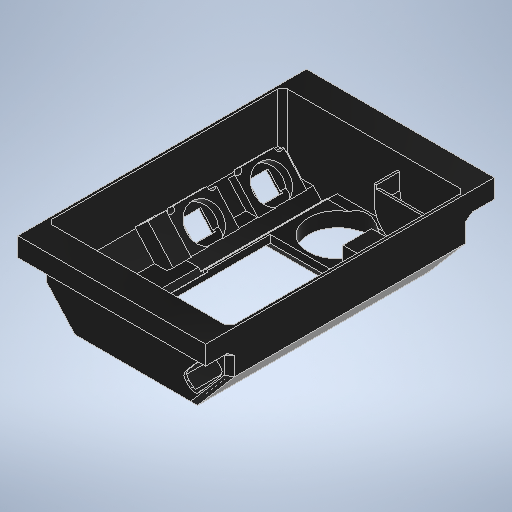
# Autodesk Inventor part: CaseTop
Saved by Autodesk Inventor 2025.2 (Build 292293000, 293)
## iProperties
Created: 2026-02-20
Part Number: CaseTop
Material: 一般
Document SubType Name: Modeling
Designer: naka6
Density: 1 g/cm^3
Appearance: ポリカーボネート - スモーク
Author: naka6
Autodesk Inventor part; units mm, degrees
ref_plane "YZ Plane" through (0, 0, 0) normal (1, 0, 0) x (0, 1, 0)
ref_plane "XZ Plane" through (0, 0, 0) normal (0, 1, 0) x (-1, 0, 0)
ref_plane "XY Plane" through (0, 0, 0) normal (0, 0, 1) x (1, 0, 0)
sketch "スケッチ1" plane through (0, 0, 0) normal (0, 0, 1) x (1, 0, 0)
  line L0 (0, 0) -> (25, 0) projected
  line L1 (25, 0) -> (25, 5) projected
  line L2 (0, 5) -> (25, 5) projected
  line L3 (0, 0) -> (0, 5) projected
  line L4 (26.3508, -9.3108) -> (30.8534, -4.0296) projected
  line L5 (-3.8505, -8.7712) -> (-2.8623, -9.8668) projected
  line L6 (-1.1891, -11.7217) -> (-2.8623, -9.8668) projected
  line L7 (-1.1891, -11.7217) -> (-0.2009, -12.8172) projected
  line L8 (5.9822, -13) -> (17.9822, -13) projected
  line L9 (32.9146, -13) -> (-6.6069, -13)
  line L10 (-6.6069, -13) -> (-6.6069, 5)
  line L11 (-6.6069, 5) -> (32.9146, 5)
  line L12 (32.9146, 5) -> (32.9146, -13)
  line L13 (31.9146, 2.3326) -> (30.7123, 3.3577) projected
  line L14 (31.9222, 2.3261) -> (31.4032, 1.7173) projected
  line L15 (-3.3792, -0.7537) -> (-5.6069, -2.7631) projected
  line L16 (-4.6007, -5.2223) -> (0.0879, -10.4201) projected
  line L17 (32.9146, -4) -> (24.3535, -14.0417)
  line L18 (-0.036, -13) -> (-6.6069, -5.7154)
  point P0 (-5.6069, -7.8692)
  point P1 (25.2416, -13)
  dimension "d0" = 0
  dimension "d1" = 0
  dimension "d2" = 0
  dimension "d26" = 1
  dimension "d27" = 1
  constraints: 12 end point, 4 parallel, 2 point on line, 1 horizontal, 1 midpoint, 1 perpendicular
  measures "d0" distance between parallel lines of L11 L2
  measures "d1" distance between parallel lines of L9 L8
  measures "d2" distance between parallel lines of L18 L6
  measures "d26" distance from line of L12 L13.start
  measures "d27" distance from line of L10 L15.end
extrude "押し出し1" add sketch "スケッチ1" along normal blind 1 contours L3 L2 L1 L0 | L0 L1 L11 L12 L17 L9 L8 L18 L7 L6 L5 L10 L3
sketch "スケッチ2" plane through (0, 0, 0) normal (0, 0, -1) x (-1, 0, 0)
  line L0 (6.6069, 5) -> (6.6069, -5.7154) projected
  line L1 (-32.9146, 5) -> (6.6069, 5) projected
  line L2 (-32.9146, -4) -> (-32.9146, 5) projected
  line L3 (0.036, -13) -> (-25.2416, -13) projected
  line L4 (-25.2416, -13) -> (-32.9146, -4) projected
  line L5 (6.6069, -5.7154) -> (0.036, -13) projected
  point P0 (0, 0)
extrude "押し出し2" add sketch "スケッチ2" along normal blind 49.75
shell "シェル1" thickness 0.6 removed faces 1 at (19.7408, 5, -15.9167)
sketch "スケッチ3" plane through (0.2308, -12.4, -49.15) normal (0, 1, 0) x (1, 0, 0)
  circle A0 centre (15.0015, -6.4) radius 0.25 projected
  circle A1 centre (8.5015, -6.4) radius 0.25 projected
  circle A2 centre (11.7515, -6.4) radius 6 projected
  line L0 (18.7692, -13.65) -> (18.7692, -44.15) construction
  line L1 (4.7692, -13.65) -> (18.7692, -13.65) construction
  line L2 (17.8672, -13.65) -> (17.8672, -44.15) construction
  line L3 (4.7692, -44.15) -> (4.7692, -13.65) construction
  line L4 (18.7692, -44.15) -> (4.7692, -44.15) construction
  circle A3 centre (11.7515, -6.4) radius 6.2
  point P0 (-0.2308, -49.15)
  dimension "d22" = 0.2
  constraints: 1 centre point
  measures "d22" radial gap between concentric circles of A2 A3
extrude "押し出し3" cut sketch "スケッチ3" against normal through all contours A0 | A1 | A2 | A3
sketch "スケッチ4" plane through (-0.036, -13, 1) normal (0, -1, 0) x (1, 0, 0)
  line L0 (19.036, -36.5) -> (19.036, -6) projected
  line L1 (5.036, -36.5) -> (19.036, -36.5) projected
  line L2 (5.036, -6) -> (5.036, -36.5) projected
  line L3 (19.036, -6) -> (5.036, -6) projected
  line L4 (19.236, -5.8) -> (19.236, -36.7)
  line L5 (19.236, -36.7) -> (4.836, -36.7)
  line L6 (4.836, -36.7) -> (4.836, -5.8)
  line L7 (4.836, -5.8) -> (19.236, -5.8)
  point P0 (0.036, -1)
  dimension "d12" = 0.2
  constraints: 8 end point, 3 other
  measures "d12" distance between parallel lines of L0 L4
extrude "押し出し4" cut sketch "スケッチ4" against normal through all contours L1 L2 L3 L0 | L4 L5 L6 L7
sketch "スケッチ5" plane through (0.2308, -12.4, -49.15) normal (0, 1, 0) x (1, 0, 0)
  line L0 (24.7339, 0) -> (24.7339, -49.55) projected
  line L1 (24.7339, 0) -> (0, 0) projected
  line L2 (0, 0) -> (0, -49.55) projected
  line L3 (0, -49.55) -> (24.7339, -49.55) projected
  line L4 (18.9692, -13.45) -> (4.5692, -13.45) projected
  line L5 (4.5692, -13.45) -> (4.5692, -44.35) projected
  line L6 (4.5692, -44.35) -> (18.9692, -44.35) projected
  line L7 (18.9692, -44.35) -> (18.9692, -13.45) projected
  circle A0 centre (11.7515, -6.4) radius 6.2 projected
  line L8 (25.0108, 0.6) -> (25.0108, -50.15) projected
  line L9 (-0.2668, -50.15) -> (25.0108, -50.15) projected
  line L10 (-0.2668, 0.6) -> (-0.2668, -50.15) projected
  line L11 (25.0108, 0.6) -> (-0.2668, 0.6) projected
  point P0 (-0.2308, -49.15)
extrude "押し出し5" add sketch "スケッチ5" along normal blind 2.5 contours L0 L3 L2 L1
chamfer "面取り1" distance 2.5 distance2 1.5 3 edges at (4.8, -13, -20.25) (12, -13, -4.8) (19.2, -13, -20.25) measured on face at (4.3, -13, -20.25) measured on face at (12, -13, -4.3) measured on face at (19.7, -13, -20.25)
chamfer "面取り3" distance 0.6 distance2 1.5 3 edges at (3.55, -13, -35.7) (12, -13, -35.7) (20.45, -13, -35.7) measured on face at (3.55, -13, -36.2) measured on face at (20.45, -13, -36.2) measured on face at (12, -13, -36.2)
sketch "スケッチ7" plane through (-0.036, -13, -49.75) normal (-0.7425471, -0.6697938, 0) x (0, 0, 1)
  line L0 (23.2879, 7.2327) -> (19.4879, 7.2327) projected
  line L1 (19.4879, 7.2327) -> (19.4879, 3.4327) projected
  line L2 (19.4879, 3.4327) -> (23.2879, 3.4327) projected
  line L3 (23.2879, 3.4327) -> (23.2879, 7.2327) projected
  circle A0 centre (21.3879, 5.3327) radius 0.9 projected
  line L4 (9.1216, 7.2327) -> (5.3216, 7.2327) projected
  line L5 (5.3216, 7.2327) -> (5.3216, 3.4327) projected
  line L6 (5.3216, 3.4327) -> (9.1216, 3.4327) projected
  line L7 (9.1216, 3.4327) -> (9.1216, 7.2327) projected
  circle A1 centre (7.2216, 5.3327) radius 0.9 projected
  line L8 (23.4879, 7.4327) -> (19.2879, 7.4327)
  line L9 (19.2879, 7.4327) -> (19.2879, 3.2327)
  line L10 (19.2879, 3.2327) -> (23.4879, 3.2327)
  line L11 (23.4879, 3.2327) -> (23.4879, 7.4327)
  line L12 (9.3216, 7.4327) -> (5.1216, 7.4327)
  line L13 (5.1216, 7.4327) -> (5.1216, 3.2327)
  line L14 (5.1216, 3.2327) -> (9.3216, 3.2327)
  line L15 (9.3216, 3.2327) -> (9.3216, 7.4327)
  point P0 (49.75, 9.629)
  dimension "d30" = 0.2
  dimension "d31" = 0.2
  constraints: 16 end point, 6 other
  measures "d30" distance between parallel lines of L3 L11
  measures "d31" distance between parallel lines of L7 L15
sketch "スケッチ8" plane through (24.9647, -12.4, -49.15) normal (1, 0, 0) x (0, 0, -1)
  line L0 (0, 0) -> (-49.55, 0) projected
  line L1 (0, 2.5) -> (0, 0) projected
  line L2 (-49.55, 2.5) -> (0, 2.5) projected
  line L3 (-49.55, 0) -> (-49.55, 2.5) projected
  point P0 (-49.15, 12.4)
extrude "押し出し8" add sketch "スケッチ8" along normal up to surface surface through (24.785, -12.6107, 0) normal (0.7609777, -0.6487781, 0)
sketch "スケッチ9" plane through (0.2308, -12.4, 0.4) normal (-1, 0, 0) x (0, 0, 1)
  line L0 (-49.55, 0) -> (0, 0) projected
  line L1 (0, 2.5) -> (0, 0) projected
  line L2 (-49.55, 2.5) -> (0, 2.5) projected
  line L3 (-49.55, 0) -> (-49.55, 2.5) projected
  point P0 (-0.4, 12.4)
extrude "押し出し9" add sketch "スケッチ9" along normal up to surface surface through (-6.1613, -5.3136, 0) normal (-0.7425471, -0.6697938, 0)
extrude "押し出し10" cut sketch "スケッチ7" against normal through all contours L3 L2 L1 L0 | A0 | L7 L6 L5 L4 | A1 | L11 L10 L9 L8 | L15 L14 L13 L12
sketch "スケッチ10" plane through (-0.036, -13, -49.75) normal (-0.7425471, -0.6697938, 0) x (0, 0, 1)
  arc A0 (41.0449, 0.0976) -> (43.25, 1.686) centre (40.65, 2.9706) ccw projected
  arc A1 (40.8745, 0.2462) -> (41.0449, 0.0976) centre (41.0245, 0.2462) ccw projected
  arc A2 (40.8745, 0.2462) -> (40.4255, 0.2462) centre (40.65, 0.2463) ccw projected
  line L0 (9.3216, 3.2327) -> (5.1216, 3.2327) projected
  line L1 (5.1216, 3.2327) -> (5.1216, 7.4327) projected
  line L2 (5.1216, 7.4327) -> (9.3216, 7.4327) projected
  line L3 (9.3216, 7.4327) -> (9.3216, 3.2327) projected
  line L4 (23.4879, 3.2327) -> (19.2879, 3.2327) projected
  line L5 (19.2879, 3.2327) -> (19.2879, 7.4327) projected
  line L6 (19.2879, 7.4327) -> (23.4879, 7.4327) projected
  line L7 (23.4879, 7.4327) -> (23.4879, 3.2327) projected
  line L8 (0, 0) -> (50.75, 0) projected
  line L9 (50.75, 9.8102) -> (50.75, 0) projected
  line L10 (0, 9.8102) -> (50.75, 9.8102) projected
  line L11 (0, 0) -> (0, 9.8102) projected
  arc A3 (40.2551, 0.0976) -> (40.4255, 0.2462) centre (40.2755, 0.2462) ccw projected
  arc A4 (38.05, 1.686) -> (40.2551, 0.0976) centre (40.65, 2.9706) ccw projected
  line L12 (43.25, 1.686) -> (43.25, 4.2551) projected
  arc A5 (43.25, 4.2551) -> (41.0449, 5.8435) centre (40.65, 2.9706) ccw projected
  line L13 (38.05, 4.2551) -> (38.05, 1.686) projected
  arc A6 (40.2551, 5.8435) -> (38.05, 4.2551) centre (40.65, 2.9706) ccw projected
  arc A7 (40.4255, 5.6949) -> (40.2551, 5.8435) centre (40.2755, 5.6949) ccw projected
  arc A8 (40.4255, 5.6949) -> (40.8745, 5.6949) centre (40.65, 5.6949) ccw projected
  arc A9 (41.0449, 5.8435) -> (40.8745, 5.6949) centre (41.0245, 5.6949) ccw projected
  point P0 (49.75, 9.629)
  point P1 (40.4255, 0.2462)
extrude "押し出し11" cut sketch "スケッチ10" against normal through all contours A1 A2 A3 A4 L13 A6 A7 A8 A9 A5 L12 A0
sketch "スケッチ11" plane through (-6.0069, -5.4848, 0.4) normal (0.7425471, 0.6697938, 0) x (0, 0, -1)
  line L0 (6.9, -5.3245) -> (6.9, -7.8936) projected
  arc A0 (6.9, -7.8936) -> (9.1051, -9.482) centre (9.5, -6.609) ccw projected
  arc A1 (9.1051, -9.482) -> (9.2755, -9.3334) centre (9.1255, -9.3334) ccw projected
  arc A2 (9.7245, -9.3334) -> (9.2755, -9.3334) centre (9.5, -9.3333) ccw projected
  arc A3 (9.7245, -9.3334) -> (9.8949, -9.482) centre (9.8745, -9.3334) ccw projected
  arc A4 (9.8949, -9.482) -> (12.1, -7.8936) centre (9.5, -6.609) ccw projected
  line L1 (12.1, -7.8936) -> (12.1, -5.3245) projected
  arc A5 (12.1, -5.3245) -> (9.8949, -3.736) centre (9.5, -6.609) ccw projected
  arc A6 (9.8949, -3.736) -> (9.7245, -3.8846) centre (9.8745, -3.8846) ccw projected
  arc A7 (9.2755, -3.8847) -> (9.7245, -3.8846) centre (9.5, -3.8847) ccw projected
  arc A8 (9.2755, -3.8847) -> (9.1051, -3.736) centre (9.1255, -3.8846) ccw projected
  arc A9 (9.1051, -3.736) -> (6.9, -5.3245) centre (9.5, -6.609) ccw projected
  line L2 (40.8284, -6.3469) -> (45.0284, -6.3469) projected
  line L3 (45.0284, -6.3469) -> (45.0284, -2.1469) projected
  line L4 (45.0284, -2.1469) -> (40.8284, -2.1469) projected
  line L5 (40.8284, -2.1469) -> (40.8284, -6.3469) projected
  line L6 (26.6621, -6.3469) -> (30.8621, -6.3469) projected
  line L7 (30.8621, -6.3469) -> (30.8621, -2.1469) projected
  line L8 (30.8621, -2.1469) -> (26.6621, -2.1469) projected
  line L9 (26.6621, -2.1469) -> (26.6621, -6.3469) projected
  line L10 (50.15, -9.5796) -> (-0.6, -9.5796) projected
  line L11 (-0.6, 0.2306) -> (-0.6, -9.5796) projected
  line L12 (50.15, 0.2306) -> (-0.6, 0.2306) projected
  line L13 (50.15, -9.5796) -> (50.15, 0.2306) projected
  circle A10 centre (42.9284, -4.2469) radius 3.5 projected
  line L14 (23.2621, -9.0398) -> (23.2621, 0.546) projected
  line L15 (23.2621, 0.546) -> (23.9692, 1.2531) projected
  line L16 (23.9692, 1.2531) -> (33.555, 1.2531) projected
  line L17 (33.555, 1.2531) -> (34.2621, 0.546) projected
  line L18 (34.2621, 0.546) -> (34.2621, -9.0398) projected
  line L19 (34.2621, -9.0398) -> (33.555, -9.7469) projected
  line L20 (33.555, -9.7469) -> (23.9692, -9.7469) projected
  line L21 (23.9692, -9.7469) -> (23.2621, -9.0398) projected
  circle A11 centre (28.7621, -4.2469) radius 3.5 projected
  circle A12 centre (33.1621, -8.6469) radius 0.7 projected
  circle A13 centre (24.3621, -8.6469) radius 0.7 projected
  circle A14 centre (24.3621, 0.1531) radius 0.7 projected
  circle A15 centre (33.1621, 0.1531) radius 0.7 projected
  line L22 (37.4284, -9.0398) -> (37.4284, 0.546) projected
  line L23 (37.4284, 0.546) -> (38.1355, 1.2531) projected
  line L24 (38.1355, 1.2531) -> (47.7213, 1.2531) projected
  line L25 (47.7213, 1.2531) -> (48.4284, 0.546) projected
  line L26 (48.4284, 0.546) -> (48.4284, -9.0398) projected
  line L27 (48.4284, -9.0398) -> (47.7213, -9.7469) projected
  line L28 (47.7213, -9.7469) -> (38.1355, -9.7469) projected
  line L29 (38.1355, -9.7469) -> (37.4284, -9.0398) projected
  circle A16 centre (42.9284, -4.2469) radius 3.5 projected
  circle A17 centre (47.3284, -8.6469) radius 0.7 projected
  circle A18 centre (38.5284, -8.6469) radius 0.7 projected
  circle A19 centre (38.5284, 0.1531) radius 0.7 projected
  circle A20 centre (47.3284, 0.1531) radius 0.7 projected
  line L30 (22.4, 0.2429) -> (22.4, -10.7571) projected
  line L31 (22.4, -10.7571) -> (0.4, -10.7571) projected
  line L32 (0.4, -10.7571) -> (0.4, 0.2429) projected
  line L33 (0.4, 0.2429) -> (22.4, 0.2429) projected
  line L34 (19.8649, -8.2571) -> (20.8649, -8.2571) projected
  arc A21 (19.8649, -8.2571) -> (19.8649, -10.2571) centre (19.8649, -9.2571) ccw projected
  line L35 (20.8649, -10.2571) -> (19.8649, -10.2571) projected
  arc A22 (20.8649, -10.2571) -> (20.8649, -8.2571) centre (20.8649, -9.2571) ccw projected
  line L36 (19.8649, -4.2571) -> (20.8649, -4.2571) projected
  arc A23 (19.8649, -4.2571) -> (19.8649, -6.2571) centre (19.8649, -5.2571) ccw projected
  line L37 (20.8649, -6.2571) -> (19.8649, -6.2571) projected
  arc A24 (20.8649, -6.2571) -> (20.8649, -4.2571) centre (20.8649, -5.2571) ccw projected
  line L38 (1.6, -0.2571) -> (2.6, -0.2571) projected
  arc A25 (1.6, -0.2571) -> (1.6, -2.2571) centre (1.6, -1.2571) ccw projected
  line L39 (2.6, -2.2571) -> (1.6, -2.2571) projected
  arc A26 (2.6, -2.2571) -> (2.6, -0.2571) centre (2.6, -1.2571) ccw projected
  line L40 (1.6, -8.2571) -> (2.6, -8.2571) projected
  arc A27 (1.6, -8.2571) -> (1.6, -10.2571) centre (1.6, -9.2571) ccw projected
  line L41 (2.6, -10.2571) -> (1.6, -10.2571) projected
  arc A28 (2.6, -10.2571) -> (2.6, -8.2571) centre (2.6, -9.2571) ccw projected
  line L42 (24.1349, -9.3469) -> (33.3893, -9.3469)
  line L43 (33.3893, -9.3469) -> (33.8621, -8.8741)
  line L44 (33.8621, -8.8741) -> (33.8621, 0.3803)
  line L45 (33.8621, 0.3803) -> (33.3893, 0.8531)
  line L46 (33.3893, 0.8531) -> (24.1349, 0.8531)
  line L47 (24.1349, 0.8531) -> (23.6621, 0.3803)
  line L48 (23.6621, 0.3803) -> (23.6621, -8.8741)
  line L49 (23.6621, -8.8741) -> (24.1349, -9.3469)
  circle A29 centre (24.3621, -8.6469) radius 0.9
  circle A30 centre (33.1621, -8.6469) radius 0.9
  circle A31 centre (33.1621, 0.1531) radius 0.9
  circle A32 centre (24.3621, 0.1531) radius 0.9
  circle A33 centre (28.7621, -4.2469) radius 3.7
  line L50 (38.3012, -9.3469) -> (47.5556, -9.3469)
  line L51 (47.5556, -9.3469) -> (48.0284, -8.8741)
  line L52 (48.0284, -8.8741) -> (48.0284, 0.3803)
  line L53 (48.0284, 0.3803) -> (47.5556, 0.8531)
  line L54 (47.5556, 0.8531) -> (38.3012, 0.8531)
  line L55 (38.3012, 0.8531) -> (37.8284, 0.3803)
  line L56 (37.8284, 0.3803) -> (37.8284, -8.8741)
  line L57 (37.8284, -8.8741) -> (38.3012, -9.3469)
  circle A34 centre (38.5284, -8.6469) radius 0.9
  circle A35 centre (38.5284, 0.1531) radius 0.9
  circle A36 centre (47.3284, 0.1531) radius 0.9
  circle A37 centre (47.3284, -8.6469) radius 0.9
  circle A38 centre (42.9284, -4.2469) radius 3.7
  line L58 (22.4, -10.7571) -> (18.6046, -10.7571)
  line L59 (18.6046, -10.7571) -> (18.6046, 0.2429)
  line L60 (18.6046, 0.2429) -> (22.4, 0.2429)
  line L61 (22.4, 0.2429) -> (22.4, -10.7571)
  line L62 (0.4, -10.7571) -> (3.8976, -10.7571)
  line L63 (3.8976, -10.7571) -> (3.8976, -7.8936)
  line L64 (3.8976, -7.8936) -> (0.4, -7.8936)
  line L65 (0.4, -7.8936) -> (0.4, -10.7571)
  line L66 (0.4, 0.0494) -> (3.8976, 0.0494)
  line L67 (3.8976, 0.0494) -> (3.8976, -2.666)
  line L68 (3.8976, -2.666) -> (0.4, -2.666)
  line L69 (0.4, -2.666) -> (0.4, 0.0494)
  point P0 (46.7627, -9.3469)
  point P1 (48.0284, -8.0812)
  point P2 (48.0284, -0.4126)
  point P3 (46.4318, 0.2306)
  point P4 (39.4251, 0.2306)
  point P5 (37.8284, -0.4126)
  point P6 (37.8284, -8.0812)
  point P7 (39.0941, -9.3469)
  point P8 (25.2587, 0.2306)
  point P9 (23.6621, -0.4126)
  point P10 (23.6621, -8.0812)
  point P11 (24.9278, -9.3469)
  point P12 (32.5964, -9.3469)
  point P13 (33.8621, -8.0812)
  point P14 (33.8621, -0.4126)
  point P15 (32.2654, 0.2306)
  point P16 (22.4, -9.5796)
  point P17 (22.4, 0.2306)
  point P18 (18.6046, 0.2306)
  point P19 (18.6046, -9.5796)
  point P20 (3.8976, -9.5796)
  point P21 (0.4, -7.8936)
  point P22 (0.4, -9.5796)
  point P23 (0.4, -2.666)
  dimension "d42" = 0.4
  dimension "d43" = 0.2
  dimension "d44" = 0.2
  dimension "d45" = 0.2
  dimension "d46" = 0.2
  dimension "d47" = 0.2
  dimension "d48" = 0.4
  dimension "d49" = 0.2
  dimension "d50" = 0.2
  dimension "d51" = 0.2
  dimension "d52" = 0.2
  dimension "d53" = 0.2
  constraints: 56 end point, 10 centre point, 6 parallel, 3 horizontal, 3 perpendicular, 2 point on line, 14 other
  measures "d42" distance between parallel lines of L20 L42
  measures "d43" radial gap between concentric circles of A13 A29
  measures "d44" radial gap between concentric circles of A12 A30
  measures "d45" radial gap between concentric circles of A15 A31
  measures "d46" radial gap between concentric circles of A14 A32
  measures "d47" radial gap between concentric circles of A11 A33
  measures "d48" distance between parallel lines of L28 L50
  measures "d49" radial gap between concentric circles of A18 A34
  measures "d50" radial gap between concentric circles of A19 A35
  measures "d51" radial gap between concentric circles of A20 A36
  measures "d52" radial gap between concentric circles of A17 A37
  measures "d53" radial gap between concentric circles of A16 A38
extrude "押し出し12" add sketch "スケッチ11" along normal blind 1.92 contours L10 A22 L34 A21 L59 L12 L30 | L52 A37 L50 A34 L56 A35 L12 A36 | L10 A21 L34 A22 | A32 L12 A31 L44 A30 L42 A29 L48 | L10 A28 L40 A27 L32 L64 L63 | L66 L67 L68 L32 | L10 A27 L40 A28 | L36 A24 L37 A23 | L38 A26 L39 A25
sketch "スケッチ12" plane through (-4.5812, -4.1988, 0.4) normal (0.7425471, 0.6697938, 0) x (0, 0, -1)
  line L0 (22.4, -7.6779) -> (18.6046, -7.6779) projected
  line L1 (22.4, -7.6779) -> (22.4, 0.2306) projected
  line L2 (22.4, 0.2306) -> (18.6046, 0.2306) projected
  line L3 (18.6046, 0.2306) -> (18.6046, -7.6779) projected
  line L4 (3.8976, 0.0494) -> (0.4, 0.0494) projected
  line L5 (0.4, 0.0494) -> (0.4, -2.666) projected
  line L6 (0.4, -2.666) -> (3.8976, -2.666) projected
  line L7 (3.8976, -2.666) -> (3.8976, 0.0494) projected
  point P0 (0.4, 0.0494)
extrude "押し出し13" add sketch "スケッチ12" along normal blind 1.8
sketch "スケッチ13" plane through (32.3146, 5, 0.4) normal (0, 0, -1) x (-1, 0, 0)
  line L0 (28.2057, -15.8469) -> (27.3146, -15.0431) projected
  line L1 (35.5734, -7.6788) -> (28.2057, -15.8469) projected
  line L2 (27.3146, -15.0431) -> (27.156, -14.9)
  line L3 (5.2186, -14.9) -> (34.3389, -14.9) projected
  point P0 (32.3146, -5)
  point P1 (29.0597, -14.9)
  constraints: 2 end point, 1 collinear, 1 point on line
extrude "押し出し14" cut sketch "スケッチ13" along normal blind 23
sketch "スケッチ14" plane through (-6.0069, 5, -49.15) normal (0, 0, 1) x (1, 0, 0)
  line L0 (0.4, -7.7631) -> (1.0698, -8.5057)
  line L1 (2.6276, -5.7537) -> (0.4, -7.7631)
  line L2 (7.7677, -15.9311) -> (1.0698, -8.5057)
  line L3 (7.7677, -15.9311) -> (9.9954, -13.9218)
  line L4 (3.9826, -14.9) -> (33.1029, -14.9)
  line L5 (6.6742, -15.1668) -> (7.6119, -16.2063)
  line L6 (5.8059, -17.8172) -> (9.04, -14.9)
  line L7 (6.6742, -15.1668) -> (6.4336, -14.9)
  line L8 (8.4375, -16.6737) -> (7.7677, -15.9311)
  line L9 (10.6652, -14.6643) -> (8.4375, -16.6737)
  line L10 (8.4375, -16.6737) -> (6.9671, -18)
  line L11 (5.9708, -18) -> (31.2484, -18)
  line L12 (7.6029, -16.1963) -> (8.2148, -16.8746)
  point P0 (6.0069, -5)
  point P1 (7.6029, -16.1963)
  point P2 (10.4039, -14.9)
extrude "押し出し15" cut sketch "スケッチ14" along normal blind 27
sketch "スケッチ15" plane through (32.3146, 5, 0.4) normal (0, 0, -1) x (-1, 0, 0)
  line L0 (12.0704, -16.3714) -> (11.5514, -15.7627) projected
  line L1 (0.9114, -3.2827) -> (11.5514, -15.7627) projected
  line L2 (13.2804, -15.3399) -> (12.078, -16.365) projected
  line L3 (13.2804, -15.3399) -> (13.7964, -14.9)
  line L4 (27.9176, -14.9) -> (5.2186, -14.9) projected
  line L5 (12.078, -16.365) -> (12.0704, -16.3714)
  point P0 (32.3146, -5)
  point P1 (10.8159, -14.9)
  constraints: 4 end point, 1 collinear, 1 point on line
extrude "押し出し16" cut sketch "スケッチ15" along normal blind 25.25
sketch "スケッチ16" plane through (0, 0, 1) normal (0, 0, 1) x (1, 0, 0)
  line L0 (26.3508, -9.3108) -> (30.8534, -4.0296) projected
  arc A0 (24.9411, -9.423) -> (26.3508, -9.3108) centre (25.5899, -8.662) ccw projected
  line L1 (24.0203, -8.638) -> (24.9411, -9.423) projected
  arc A1 (30.8534, -4.0296) -> (30.7412, -2.6198) centre (30.0924, -3.3808) ccw projected
  line L2 (30.7412, -2.6198) -> (29.8204, -1.8348) projected
  arc A2 (29.8204, -1.8348) -> (28.4106, -1.947) centre (29.1716, -2.5958) ccw projected
  line L3 (28.4106, -1.947) -> (25.9323, -4.854) projected
  line L4 (25.8998, -4.892) -> (23.9081, -7.2282) projected
  arc A3 (23.9081, -7.2282) -> (24.0203, -8.638) centre (24.6691, -7.877) ccw projected
  line L5 (25.6716, -4.6974) -> (23.6798, -7.0336)
  arc A4 (23.6798, -7.0336) -> (23.8257, -8.8663) centre (24.6691, -7.877) ccw
  line L6 (23.8257, -8.8663) -> (24.7464, -9.6513)
  arc A5 (24.7464, -9.6513) -> (26.5791, -9.5054) centre (25.5899, -8.662) ccw
  line L7 (26.5791, -9.5054) -> (31.0817, -4.2242)
  arc A6 (31.0817, -4.2242) -> (30.9358, -2.3916) centre (30.0924, -3.3808) ccw
  line L8 (30.9358, -2.3916) -> (30.015, -1.6065)
  arc A7 (30.015, -1.6065) -> (28.1823, -1.7524) centre (29.1716, -2.5958) ccw
  line L9 (28.1823, -1.7524) -> (25.704, -4.6593)
  line L10 (25.6716, -4.6974) -> (25.704, -4.6593)
  point P0 (0, 0)
  dimension "d64" = 0.3
  constraints: 12 end point, 8 point on circle, 4 centre point, 1 collinear, 8 other
  measures "d64" distance between parallel lines of L4 L5
extrude "押し出し17" cut sketch "スケッチ16" against normal blind 8
sketch "スケッチ17" plane through (32.3146, -3.7789, -49.15) normal (-0.7609777, 0.6487781, 0) x (0, 0, 1)
  line L0 (0, 0) -> (49.55, 0) projected
  line L1 (0, -8.0437) -> (49.55, -8.0437) projected
  arc A0 (48.1, 3.5912) -> (47.31, 4.3912) centre (47.3, 3.5912) ccw projected
  line L2 (47.31, 4.3912) -> (47.31, 3.0112) projected
  arc A1 (45.71, 3.0112) -> (47.31, 3.0112) centre (46.51, 3.0112) ccw projected
  line L3 (45.71, 3.0112) -> (45.71, 4.3912) projected
  line L4 (45.71, 4.3912) -> (44.77, 4.3912) projected
  line L5 (44.77, 4.3912) -> (44.77, 3.0112) projected
  arc A2 (43.17, 3.0112) -> (44.77, 3.0112) centre (43.97, 3.0112) ccw projected
  line L6 (43.17, 3.0112) -> (43.17, 4.3912) projected
  line L7 (43.17, 4.3912) -> (42.23, 4.3912) projected
  line L8 (42.23, 4.3912) -> (42.23, 3.0112) projected
  arc A3 (40.63, 3.0112) -> (42.23, 3.0112) centre (41.43, 3.0112) ccw projected
  line L9 (40.63, 3.0112) -> (40.63, 4.3912) projected
  line L10 (40.63, 4.3912) -> (39.69, 4.3912) projected
  line L11 (39.69, 4.3912) -> (39.69, 3.0112) projected
  arc A4 (38.09, 3.0112) -> (39.69, 3.0112) centre (38.89, 3.0112) ccw projected
  line L12 (38.09, 3.0112) -> (38.09, 4.3912) projected
  line L13 (38.09, 4.3912) -> (37.15, 4.3912) projected
  line L14 (37.15, 4.3912) -> (37.15, 3.0112) projected
  arc A5 (35.55, 3.0112) -> (37.15, 3.0112) centre (36.35, 3.0112) ccw projected
  line L15 (35.55, 3.0112) -> (35.55, 4.3912) projected
  line L16 (35.55, 4.3912) -> (34.61, 4.3912) projected
  line L17 (34.61, 4.3912) -> (34.61, 3.0112) projected
  arc A6 (33.01, 3.0112) -> (34.61, 3.0112) centre (33.81, 3.0112) ccw projected
  line L18 (33.01, 3.0112) -> (33.01, 4.3912) projected
  line L19 (33.01, 4.3912) -> (32.07, 4.3912) projected
  line L20 (32.07, 4.3912) -> (32.07, 3.0112) projected
  arc A7 (30.47, 3.0112) -> (32.07, 3.0112) centre (31.27, 3.0112) ccw projected
  line L21 (30.47, 3.0112) -> (30.47, 4.3912) projected
  line L22 (30.47, 4.3912) -> (29.53, 4.3912) projected
  line L23 (29.53, 4.3912) -> (29.53, 3.0112) projected
  arc A8 (27.93, 3.0112) -> (29.53, 3.0112) centre (28.73, 3.0112) ccw projected
  line L24 (27.93, 3.0112) -> (27.93, 4.3912) projected
  line L25 (27.93, 4.3912) -> (26.99, 4.3912) projected
  line L26 (26.99, 4.3912) -> (26.99, 3.0112) projected
  arc A9 (25.39, 3.0112) -> (26.99, 3.0112) centre (26.19, 3.0112) ccw projected
  line L27 (25.39, 3.0112) -> (25.39, 4.3912) projected
  arc A10 (25.39, 4.3912) -> (24.6, 3.5912) centre (25.4, 3.5912) ccw projected
  line L28 (24.6, 3.5912) -> (24.6, -12.8088) projected
  arc A11 (24.6, -12.8088) -> (25.39, -13.6087) centre (25.4, -12.8088) ccw projected
  line L29 (25.39, -13.6087) -> (25.39, -12.2288) projected
  arc A12 (26.99, -12.2288) -> (25.39, -12.2288) centre (26.19, -12.2288) ccw projected
  line L30 (26.99, -12.2288) -> (26.99, -13.6088) projected
  line L31 (26.99, -13.6088) -> (27.93, -13.6088) projected
  line L32 (27.93, -13.6088) -> (27.93, -12.2288) projected
  arc A13 (29.53, -12.2288) -> (27.93, -12.2288) centre (28.73, -12.2288) ccw projected
  line L33 (29.53, -12.2288) -> (29.53, -13.6088) projected
  line L34 (29.53, -13.6088) -> (30.47, -13.6088) projected
  line L35 (30.47, -13.6088) -> (30.47, -12.2288) projected
  arc A14 (32.07, -12.2288) -> (30.47, -12.2288) centre (31.27, -12.2288) ccw projected
  line L36 (32.07, -12.2288) -> (32.07, -13.6088) projected
  line L37 (32.07, -13.6088) -> (33.01, -13.6088) projected
  line L38 (33.01, -13.6088) -> (33.01, -12.2288) projected
  arc A15 (34.61, -12.2288) -> (33.01, -12.2288) centre (33.81, -12.2288) ccw projected
  line L39 (34.61, -12.2288) -> (34.61, -13.6088) projected
  line L40 (34.61, -13.6088) -> (35.55, -13.6088) projected
  line L41 (35.55, -13.6088) -> (35.55, -12.2288) projected
  arc A16 (37.15, -12.2288) -> (35.55, -12.2288) centre (36.35, -12.2288) ccw projected
  line L42 (37.15, -12.2288) -> (37.15, -13.6088) projected
  line L43 (37.15, -13.6088) -> (38.09, -13.6088) projected
  line L44 (38.09, -13.6088) -> (38.09, -12.2288) projected
  arc A17 (39.69, -12.2288) -> (38.09, -12.2288) centre (38.89, -12.2288) ccw projected
  line L45 (39.69, -12.2288) -> (39.69, -13.6088) projected
  line L46 (39.69, -13.6088) -> (40.63, -13.6088) projected
  line L47 (40.63, -13.6088) -> (40.63, -12.2288) projected
  arc A18 (42.23, -12.2288) -> (40.63, -12.2288) centre (41.43, -12.2288) ccw projected
  line L48 (42.23, -12.2288) -> (42.23, -13.6088) projected
  line L49 (42.23, -13.6088) -> (43.17, -13.6088) projected
  line L50 (43.17, -13.6088) -> (43.17, -12.2288) projected
  arc A19 (44.77, -12.2288) -> (43.17, -12.2288) centre (43.97, -12.2288) ccw projected
  line L51 (44.77, -12.2288) -> (44.77, -13.6088) projected
  line L52 (44.77, -13.6088) -> (45.71, -13.6088) projected
  line L53 (45.71, -13.6088) -> (45.71, -12.2288) projected
  arc A20 (47.31, -12.2288) -> (45.71, -12.2288) centre (46.51, -12.2288) ccw projected
  line L54 (47.31, -12.2288) -> (47.31, -13.6087) projected
  arc A21 (47.31, -13.6087) -> (48.1, -12.8088) centre (47.3, -12.8088) ccw projected
  line L55 (48.1, -12.8088) -> (48.1, 3.5912) projected
  arc A22 (46.8, -9.4288) -> (46.8, -8.4288) centre (46.8, -8.9288) ccw projected
  line L56 (46.8, -9.4288) -> (46.1, -9.4288) projected
  arc A23 (46.1, -8.4288) -> (46.1, -9.4288) centre (46.1, -8.9288) ccw projected
  line L57 (46.1, -8.4288) -> (46.8, -8.4288) projected
  line L58 (43.2, -9.4288) -> (42.5, -9.4288) projected
  arc A24 (42.5, -8.4288) -> (42.5, -9.4288) centre (42.5, -8.9288) ccw projected
  line L59 (42.5, -8.4288) -> (43.2, -8.4288) projected
  arc A25 (43.2, -9.4288) -> (43.2, -8.4288) centre (43.2, -8.9288) ccw projected
  line L60 (43.2, -0.7888) -> (42.5, -0.7888) projected
  arc A26 (42.5, 0.2112) -> (42.5, -0.7888) centre (42.5, -0.2888) ccw projected
  line L61 (42.5, 0.2112) -> (43.2, 0.2112) projected
  arc A27 (43.2, -0.7888) -> (43.2, 0.2112) centre (43.2, -0.2888) ccw projected
  circle A28 centre (39.31, 0.7612) radius 0.6 projected
  circle A29 centre (37.7171, 0.7612) radius 0.6 projected
  circle A30 centre (36.1243, 0.7612) radius 0.6 projected
  circle A31 centre (34.5314, 0.7612) radius 0.6 projected
  circle A32 centre (32.9386, 0.7612) radius 0.6 projected
  circle A33 centre (31.3457, 0.7612) radius 0.6 projected
  circle A34 centre (29.7529, 0.7612) radius 0.6 projected
  circle A35 centre (28.16, 0.7612) radius 0.6 projected
  arc A36 (46.8, -0.7888) -> (46.8, 0.2112) centre (46.8, -0.2888) ccw projected
  line L62 (46.8, -0.7888) -> (46.1, -0.7888) projected
  arc A37 (46.1, 0.2112) -> (46.1, -0.7888) centre (46.1, -0.2888) ccw projected
  line L63 (46.1, 0.2112) -> (46.8, 0.2112) projected
  line L64 (24.6, 0) -> (26.99, 0)
  line L65 (26.99, 0) -> (26.99, -3.7543)
  line L66 (26.99, -3.7543) -> (24.6, -3.7543)
  line L67 (24.6, -3.7543) -> (24.6, 0)
  point P0 (49.15, -18.0893)
  point P1 (24.6, -3.7543)
  constraints: 8 end point, 2 parallel, 2 point on line, 1 horizontal, 1 perpendicular
extrude "押し出し18" add sketch "スケッチ17" along normal blind 4 contours L0 L65 L66 L28
sketch "スケッチ18" plane through (0.2308, -9.9, -49.15) normal (0, 1, 0) x (1, 0, 0)
  line L0 (18.2874, -49.55) -> (18.2874, -44.35) projected
  line L1 (18.2874, -44.35) -> (4.9279, -44.35) projected
  line L2 (4.9279, -44.35) -> (4.9279, -49.55) projected
  line L3 (18.2874, -49.55) -> (4.9279, -49.55) projected
  circle A0 centre (11.7515, -6.4) radius 6.2 projected
  line L4 (24.9624, -49.55) -> (24.9624, -42.15) projected
  line L5 (24.9624, -42.15) -> (25.7558, -42.15) projected
  line L6 (25.7558, -42.15) -> (25.7558, -49.55) projected
  line L7 (26.8653, -49.55) -> (25.7558, -49.55) projected
  line L8 (26.8653, 0) -> (26.8653, -49.55) projected
  line L9 (4.1662, 0) -> (26.8653, 0) projected
  line L10 (4.1662, 0) -> (4.1662, -26.55) projected
  line L11 (4.1662, -26.55) -> (4.5692, -26.55) projected
  line L12 (4.5692, -26.55) -> (4.5692, -13.45) projected
  line L13 (4.5692, -13.45) -> (18.9692, -13.45) projected
  line L14 (18.9692, -13.45) -> (18.9692, -24.3) projected
  line L15 (18.9692, -24.3) -> (21.268, -24.3) projected
  line L16 (21.268, -24.3) -> (21.268, -49.55) projected
  line L17 (24.9624, -49.55) -> (21.268, -49.55) projected
  line L18 (26.8653, -12.7392) -> (19.1904, -12.7392)
  line L19 (19.1904, -12.7392) -> (19.1904, -6.7025)
  line L20 (19.1904, -6.7025) -> (26.8653, -6.7025)
  line L21 (26.8653, -6.7025) -> (26.8653, -12.7392)
  point P0 (-0.2308, -49.15)
  point P1 (26.8653, -6.7025)
  constraints: 8 end point, 2 parallel, 1 horizontal, 1 perpendicular, 1 point on line
extrude "押し出し19" add sketch "スケッチ18" along normal blind 5 contours L3 L2 L1 L0 | L18 L19 L20 L8
sketch "スケッチ19" plane through (-6.0069, 5, -49.15) normal (0, 0, 1) x (1, 0, 0)
  line L0 (38.9215, 0) -> (38.9215, -9) projected
  line L1 (38.9215, -9) -> (31.2484, -18) projected
  line L2 (31.2484, -18) -> (5.9708, -18) projected
  line L3 (5.9708, -18) -> (-0.6, -10.7154) projected
  line L4 (-0.6, -10.7154) -> (-0.6, 0) projected
  line L5 (-0.6, 0) -> (38.9215, 0) projected
  circle A0 centre (29.9105, -6.7125) radius 5 projected
  circle A1 centre (29.9105, -6.7125) radius 5.25
  line L6 (35.1605, -6.7125) -> (24.6605, -6.7125)
  line L7 (24.6605, -6.7125) -> (24.6605, 0)
  line L8 (24.6605, 0) -> (35.1605, 0)
  line L9 (35.1605, 0) -> (35.1605, -6.7125)
  circle A2 centre (29.9105, -6.7125) radius 5.75
  line L10 (24.1605, 0.5) -> (24.1605, -7.2125)
  line L11 (24.1605, -7.2125) -> (35.6605, -7.2125)
  line L12 (35.6605, -7.2125) -> (35.6605, 0.5)
  line L13 (35.6605, 0.5) -> (24.1605, 0.5)
  point P0 (6.0069, -5)
  point P1 (24.1605, 0)
  point P2 (24.1605, -6.7125)
  point P3 (35.6605, -6.7125)
  point P4 (35.6605, 0)
  dimension "d71" = 0.25
  dimension "d72" = 0.5
  dimension "d73" = 0.5
  constraints: 16 end point, 4 parallel, 2 perpendicular, 2 vertical, 1 centre point, 1 horizontal, 1 point on line, 6 other
  measures "d73" distance between parallel lines of L7 L10
extrude "押し出し20" add sketch "スケッチ19" along normal blind 4.4 contours L12 A2 L9 L5 | A2 L11 A1 L9 | L7 A2 L10 L5 | A2 L11 A1 | L7 A1 L11 A2
sketch "スケッチ20" plane through (-6.0069, 5, -44.75) normal (0, 0, 1) x (1, 0, 0)
  line L0 (24.1605, 0) -> (24.1605, -6.7125) projected
  arc A0 (24.1605, -6.7125) -> (35.6605, -6.7125) centre (29.9105, -6.7125) ccw projected
  line L1 (35.6605, -6.7125) -> (35.6605, 0) projected
  line L2 (38.9215, 0) -> (-0.6, 0) projected
  point P0 (6.0069, -5)
extrude "押し出し21" add sketch "スケッチ20" along normal blind 0.5
sketch "スケッチ21" plane through (18.1536, -1.7125, -49.15) normal (-1, 0, 0) x (0, 0, 1)
  line L0 (0, 6.7125) -> (4.9, 6.7125) projected
  line L1 (4.9, 6.7125) -> (0, 6.7125)
  line L2 (0, 6.7125) -> (0, 3.4842)
  line L3 (0, 3.4842) -> (4.9, 3.4842)
  line L4 (4.9, 3.4842) -> (4.9, 6.7125)
  point P0 (49.15, 1.7125)
  constraints: 8 end point, 2 parallel, 1 horizontal, 1 perpendicular
extrude "押し出し22" cut sketch "スケッチ21" against normal blind 0.5
sketch "スケッチ22" plane through (-6.6069, 5, 1) normal (0, 1, 0) x (1, 0, 0)
  line L0 (36.2605, 50.15) -> (36.2605, 45.25) projected
  line L1 (35.7605, 50.15) -> (35.7605, 45.75) projected
  line L2 (35.7605, 45.75) -> (25.2605, 45.75) projected
  line L3 (36.2605, 45.25) -> (25.2605, 45.25) projected
  line L4 (25.2605, 50.15) -> (25.2605, 45.75) projected
  line L5 (24.7605, 45.25) -> (24.7605, 50.15) projected
  line L6 (24.7605, 45.25) -> (24.7605, 50.15) projected
  line L7 (25.2605, 45.25) -> (24.7605, 45.25) projected
  line L8 (25.2605, 45.25) -> (25.2605, 45.75) projected
  line L9 (25.2605, 50.15) -> (25.2605, 45.75) projected
  line L10 (24.7605, 50.15) -> (25.2605, 50.15) projected
  line L11 (0.6, 50.15) -> (35.7605, 50.15) projected
  line L12 (35.7605, 50.15) -> (35.7605, 45.75) projected
  line L13 (35.7605, 45.75) -> (25.2605, 45.75) projected
  line L14 (25.2605, 45.75) -> (25.2605, 45.25) projected
  line L15 (36.2605, 45.25) -> (25.2605, 45.25) projected
  line L16 (36.2605, 50.15) -> (36.2605, 45.25) projected
  line L17 (36.2605, 50.15) -> (38.9215, 50.15) projected
  line L18 (38.9215, 50.15) -> (38.9215, 0.6) projected
  line L19 (38.9215, 0.6) -> (0.6, 0.6) projected
  line L20 (0.6, 0.6) -> (0.6, 50.15) projected
  line L21 (0, 0) -> (0, 50.75) projected
  line L22 (39.5215, 0) -> (0, 0) projected
  line L23 (39.5215, 50.75) -> (39.5215, 0) projected
  line L24 (0, 50.75) -> (39.5215, 50.75) projected
  line L25 (36.2605, 50.15) -> (24.7605, 50.15) projected
  point P0 (6.6069, 1)
extrude "押し出し23" cut sketch "スケッチ22" against normal blind 4 contours L0 L3 L8 L2 L1 L25
chamfer "面取り4" distance 1 angle 45 18 edges at (-5.2287, -7.2433, 1) (-3.3564, -9.319, 1) (-2.0257, -10.7942, 1) (-0.1185, -12.9086, 1) (-0.695, -12.2694, 1) (-6.6069, -0.3577, 1) (12.6028, -13, 1) (29.0781, -8.5, 1) (32.9146, 0.5, 1) (12.6028, -13, -49.75) (29.0781, -8.5, -49.75) (32.9146, 0.5, -49.75) (-3.3214, -9.3577, -49.75) (-6.6069, -0.3577, -49.75) (-6.0069, -0.2424, -49.15) (29.7053, -6.8395, -49.15) (-6.0069, -0.2424, 0.4) (15.7465, -9.9, -49.15)
chamfer "面取り5" distance 1 angle 45 1 edges at (32.3146, 1.3812, -49.15)
chamfer "面取り6" distance 1 angle 45 1 edges at (32.3146, 0.6105, 0.4)
sketch "スケッチ23" plane through (0, 0, -49.75) normal (0, 0, -1) x (-1, 0, 0)
  line L0 (6.6069, 5) -> (5.6069, 5) projected
  line L1 (6.6069, 5) -> (-32.9146, 5)
  line L2 (-32.9146, 5) -> (-32.9146, 1)
  line L3 (-32.9146, 1) -> (6.6069, 1)
  line L4 (6.6069, 1) -> (6.6069, 5)
  line L5 (-32.9146, 5) -> (-32.9146, -4) projected
  point P0 (0, 0)
  point P1 (-13.1539, 5)
  dimension "d91" = 4
  constraints: 8 end point, 2 parallel, 1 horizontal, 1 midpoint, 1 perpendicular, 1 point on line
  measures "d91" distance from line of point (-13.154, 5) L3
extrude "押し出し24" add sketch "スケッチ23" along normal blind 5
sketch "スケッチ24" plane through (0, 0, -49.75) normal (0, 0, 1) x (1, 0, 0)
  line L0 (-5.6069, 5) -> (-5.6069, 1) projected
  line L1 (-6.6069, 5) -> (-5.6069, 5) projected
  line L2 (-6.6069, 1) -> (-6.6069, 5) projected
  line L3 (-5.6069, 1) -> (-6.6069, 1) projected
  line L4 (31.9146, 1) -> (31.9146, 5) projected
  line L5 (32.9146, 1) -> (31.9146, 1) projected
  line L6 (32.9146, 5) -> (32.9146, 1) projected
  line L7 (31.9146, 5) -> (32.9146, 5) projected
  point P0 (0, 0)
extrude "押し出し25" add sketch "スケッチ24" along normal blind 1
chamfer "面取り7" distance 1 angle 45 3 edges at (13.1539, 1, -49.75) (32.4146, 1, -49.25) (-6.1069, 1, -49.25)
sketch "スケッチ25" plane through (0, 0, 1) normal (0, 0, 1) x (1, 0, 0)
  line L0 (32.9146, 5) -> (32.9146, 1) projected
  line L1 (-6.6069, 1) -> (-6.6069, 5) projected
  line L2 (32.9146, 5) -> (-6.6069, 5)
  line L3 (-6.6069, 5) -> (-6.6069, 1)
  line L4 (-6.6069, 1) -> (32.9146, 1)
  line L5 (32.9146, 1) -> (32.9146, 5)
  point P0 (0, 0)
  dimension "d99" = 4
  constraints: 8 end point, 2 parallel, 1 horizontal, 1 perpendicular, 1 point on line
  measures "d99" distance between parallel lines of L2 L4
extrude "押し出し26" add sketch "スケッチ25" along normal blind 5
sketch "スケッチ26" plane through (0, 0, 1) normal (0, 0, -1) x (-1, 0, 0)
  line L0 (-31.9146, 5) -> (-31.9146, 1) projected
  line L1 (-32.9146, 5) -> (-31.9146, 5) projected
  line L2 (-32.9146, 1) -> (-32.9146, 5) projected
  line L3 (-31.9146, 1) -> (-32.9146, 1) projected
  line L4 (5.6069, 1) -> (5.6069, 5) projected
  line L5 (6.6069, 1) -> (5.6069, 1) projected
  line L6 (6.6069, 5) -> (6.6069, 1) projected
  line L7 (5.6069, 5) -> (6.6069, 5) projected
  point P0 (0, 0)
extrude "押し出し27" add sketch "スケッチ26" along normal blind 1
chamfer "面取り8" distance 1 angle 45 3 edges at (13.1539, 1, 1) (32.4146, 1, 0.5) (-6.1069, 1, 0.5)
